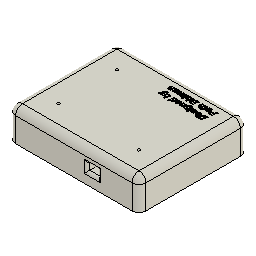
Dropsense mark-2 reciever part-1 v5 (Autodesk Fusion 360 design; units mm, degrees)
Autodesk Fusion 360 part; units mm, degrees
note: some values were not read from the file. Set by a fixed rule: which sketch regions a step uses.
sketch "Sketch1" plane through (0, 0, 0) normal (0, 0, 1) x (1, 0, 0)
  line L0 (-31.9, 24) -> (31.9, 24)
  line L1 (31.9, 24) -> (31.9, -24)
  line L2 (31.9, -24) -> (-31.9, -24)
  line L3 (-31.9, -24) -> (-31.9, 24)
  line L4 (-31.9, 24) -> (31.9, -24) construction
  line L5 (31.9, 24) -> (-31.9, -24) construction
  line L6 (-36.9, 29) -> (36.9, 29)
  line L7 (36.9, 29) -> (36.9, -29)
  line L8 (36.9, -29) -> (-36.9, -29)
  line L9 (-36.9, -29) -> (-36.9, 29)
  line L10 (-31.9, -24) -> (-28.9, -24)
  line L11 (-28.9, -24) -> (-28.9, -21)
  circle A0 centre (-28.9, -21) radius 0.95
  line L12 (0, -24) -> (0, 24)
  line L13 (-31.9, 0) -> (31.9, 0)
  circle A1 centre (28.9, -21) radius 0.95
  circle A2 centre (28.9, 21) radius 0.95
  circle A3 centre (-28.9, 21) radius 0.95
  line L14 (46.9, 39) -> (46.9, -39)
  line L15 (46.9, -39) -> (-46.9, -39)
  line L16 (-46.9, -39) -> (-46.9, 39)
  line L17 (-46.9, 39) -> (46.9, 39)
  dimension "d1" = 63.8
  dimension "d2" = 48
  dimension "d3" = -5
  dimension "d4" = 3
  dimension "d5" = 3
  dimension "d6" = 1.9
  dimension "d7" = -10
  dimension "d14" = 78
  dimension "d15" = 93.8
  constraint horizontal L0
  constraint perpendicular L0 L1
  constraint parallel L0 L2
  constraint parallel L1 L3
  constraint coincident L4 origin
  constraint coincident L5 origin
  constraint perpendicular L3 L10
  constraint coincident L2 L10.end
  constraint perpendicular L2 L11
  constraint coincident L11.end A0.centre
  constraint midpoint L0 L12.end
  constraint perpendicular L0 L12
  constraint midpoint L3 L13.start
  constraint midpoint L1 L13.end
  constraint symmetric A0 L12 A1
  constraint symmetric A0 L13 A3
  constraint symmetric L13 A1 A2
  measures "d1" distance of L1.end L2.end
  measures "d2" distance of L0.end L1.end
  measures "d4" distance of L2.end L10.end
  measures "d5" distance of L10.end L11.end
  measures "d6" diameter of A0
  measures "d14" distance of L14.start L14.end
  measures "d15" distance of L14.end L15.end
extrude "Extrude1" add sketch "Sketch1" along normal blind 10 contours L0 L3 L12 L13 | L0 L1 L12 L13 | L2 L3 L10 L12 L13 | L1 L2 L12 L13 | L6 L7 L8 L9 | L14 L15 L16 L17
extrude "Extrude2" add sketch "Sketch1" against normal blind 14.5 contours L14 L15 L16 L17
extrude "Extrude3" cut 1 faces at (-12.3, -35.6667, -14.5) along direction (0, 0, 1) blind 2
sketch "Sketch2" plane through (0, 0, 0) normal (0, 0, 1) x (1, 0, 0)
  line L0 (31.9, -22) -> (12.4, -22)
  line L1 (12.4, -22) -> (12.4, -24)
  line L2 (8.55, -24) -> (16.25, -24)
  dimension "d16" = 19.5
  dimension "d17" = 2
  dimension "d18" = 7.7
  constraint horizontal L0
  constraint perpendicular L0 L1
  constraint midpoint L1.end L2
  constraint perpendicular L1 L2
  measures "d16" distance of L0.start L0.end
  measures "d17" distance of L0.end L1.end
  measures "d18" distance of L2.start L2.end
sketch "Sketch3" plane through (0, -39, 0) normal (0, -1, 0) x (1, 0, 0)
  line L0 (-46.9, -12.5) -> (46.9, -12.5)
  line L1 (46.9, -12.5) -> (46.9, 10)
  line L2 (46.9, 10) -> (-46.9, 10)
  line L3 (-46.9, 10) -> (-46.9, -12.5)
  line L4 (9.5181, -4.304) -> (17.2181, -4.304)
  line L5 (17.2181, -4.304) -> (17.2181, 0.696)
  line L6 (17.2181, 0.696) -> (9.5181, 0.696)
  line L7 (9.5181, 0.696) -> (9.5181, -4.304)
  line L8 (9.5181, -4.304) -> (17.2181, 0.696) construction
  line L9 (17.2181, -4.304) -> (9.5181, 0.696) construction
  point P0 (13.3681, -1.804)
  dimension "d19" = 7.7
  dimension "d20" = 5
  constraint horizontal L4
  constraint perpendicular L4 L5
  constraint parallel L4 L6
  constraint parallel L5 L7
  constraint coincident L8 P0
  constraint coincident L9 P0
  measures "d19" distance of L5.end L6.end
  measures "d20" distance of L4.end L5.end
extrude "Extrude4" cut sketch "Sketch3" against normal blind 10 contours L4 L5 L6 L7
sketch "Sketch4" plane through (0, 0, -12.5) normal (0, 0, -1) x (1, 0, 0)
  line L0 (-36.9, 29) -> (36.9, 29)
  line L1 (36.9, 29) -> (36.9, -29)
  line L2 (36.9, -29) -> (-36.9, -29)
  line L3 (-36.9, -29) -> (-36.9, 29)
  line L4 (-46.9, 39) -> (-46.9, -39)
  line L5 (-46.9, -39) -> (46.9, -39)
  line L6 (46.9, -39) -> (46.9, 39)
  line L7 (46.9, 39) -> (-46.9, 39)
  line L8 (46.9, -39) -> (41.5967, -33.6967)
  line L9 (46.9, -39) -> (36.9, -39) construction
  circle A0 centre (41.5967, -33.6967) radius 1.5
  line L10 (0, -39) -> (0, 39)
  line L11 (46.9, 0) -> (-46.9, 0)
  circle A1 centre (-41.5967, -33.6967) radius 1.5
  circle A2 centre (-41.5967, 33.6967) radius 1.5
  circle A3 centre (41.5967, 33.6967) radius 1.5
  dimension "d23" = 45
  dimension "d24" = 7.5
  dimension "d25" = 3
  constraint horizontal L9
  constraint coincident L5.end L6.start
  constraint coincident L8.end A0.centre
  constraint midpoint L5 L10.start
  constraint midpoint L7 L10.end
  constraint midpoint L6 L11.start
  constraint midpoint L4 L11.end
  constraint symmetric A0 L10 A1
  constraint symmetric A0 L11 A3
  constraint symmetric L11 A1 A2
  measures "d23" angle of L8 L9
  measures "d24" distance of L5.end L8.end
  measures "d25" diameter of A0
extrude "Extrude5" cut sketch "Sketch4" against normal blind 15 contours A0 | A1 | A2 | A3
fillet "Fillet1" radius 5 4 edges at (0, 39, 10) (46.9, 0, 10) (-46.9, 0, 10) (0, -39, 10)
fillet "Fillet2" radius 5 8 edges at (-45.4355, 37.5355, 8.5355) (-46.9, 39, -3.75) (46.9, 39, -3.75) (45.4355, 37.5355, 8.5355) (46.9, -39, -3.75) (45.4355, -37.5355, 8.5355) (-46.9, -39, -3.75) (-45.4355, -37.5355, 8.5355)
fillet "Fillet3" radius 2 4 edges at (17.2181, -39, -1.804) (13.3681, -39, -4.304) (9.5181, -39, -1.804) (13.3681, -39, 0.696)
sketch "Sketch5" plane through (0, 0, 10) normal (0, 0, 1) x (-1, 0, 0)
  circle A0 centre (-28.9, -21) radius 0.95
  circle A1 centre (-28.9, 21) radius 0.95
  circle A2 centre (28.9, 21) radius 0.95
  circle A3 centre (28.9, -21) radius 0.95
  line L0 (41.9, 34) -> (-41.9, 34)
  line L1 (-41.9, 34) -> (-41.9, -34)
  line L2 (-41.9, -34) -> (41.9, -34)
  line L3 (41.9, -34) -> (41.9, 34)
  line L4 (-41.9, -34) -> (0, -34) construction
  line L5 (0, -34) -> (0, -17) construction
  line L6 (0, -17) -> (-41.9, -17) construction
  line L7 (-41.9, -17) -> (-41.9, -34) construction
  dimension "d34" = 4
  text T0 "Designed by Path Dhiman" font "Arial" height 4 bold italic align right middle in box 41.9 x 17 at (-41.9, -34) x (1, 0) y (0, 1) spacing 1
extrude "Extrude6" cut sketch "Sketch5" against normal blind 1 text T0
equation "d35 = 'Designed by Path Dhiman'"
